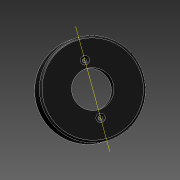
# Autodesk Inventor part: Griff01
Saved by Autodesk Inventor 2013 (Build 170138000, 138)
## iProperties
Created: 2006-09-13
Part Number: Griff01
Document SubType Name: Modeling
Designer: acad
Manufacturer: Standard
Standards Organization: Custom
Material: Allgemein
Density: 1 g/cm^3
Author: acad
Autodesk Inventor part; units mm, degrees
ref_plane "YZ Plane" through (0, 0, 0) normal (1, 0, 0) x (0, 1, 0)
ref_plane "XZ Plane" through (0, 0, 0) normal (0, 1, 0) x (-1, 0, 0)
ref_plane "XY Plane" through (0, 0, 0) normal (0, 0, 1) x (1, 0, 0)
sketch "Skizze1" plane through (0, 0, 0) normal (0, 0, 1) x (1, 0, 0)
  circle A0 centre (0, 0) radius 22.5
  circle A1 centre (0, 0) radius 9
  dimension "d0" = 45
  dimension "d2" = 9
  constraints: 2 centre point, 1 concentric
  measures "d0" diameter of A0
  measures "d2" radius of A1
extrude "Extrusion1" add sketch "Skizze1" along normal blind 15
sketch "Skizze3" plane through (0, 0, 0) normal (0, 0, -1) x (-1, 0, 0)
  circle A0 centre (0, 0) radius 9 projected
  circle A1 centre (0, 0) radius 22.5 projected
  circle A2 centre (0, 0) radius 16
  dimension "d5" = 32
  constraints: 1 centre point, 1 coincident
  measures "d5" diameter of A2
extrude "Extrusion2" cut sketch "Skizze3" against normal blind 8 contours A2
sketch "Skizze4" plane through (0, 0, 15) normal (0, 0, 1) x (1, 0, 0)
  circle A0 centre (0, 0) radius 9 projected
  circle A1 centre (0, 0) radius 16 projected
  line L0 (-27, 0) -> (36, 0) projected
  point P0 (-12.5, 0)
  point P1 (12.5, 0)
  dimension "d8" = 12.5
  dimension "d9" = 12.5
  constraints: 2 point on line
  measures "d8" distance of point (-12.5, 0) A0.centre
  measures "d9" distance of A0.centre point (12.5, 0)
hole "Bohrung1" at (-12.5, 0, 15) at (12.5, 0, 15) direction (0, 0, -1) diameter 2 end through all countersink diameter 4 countersink angle 90
fillet "Rundung1" radius 1 2 edges at (-22.5, 0, 15) (-22.5, 0, 0)
equation "\"d9\" = d8"
